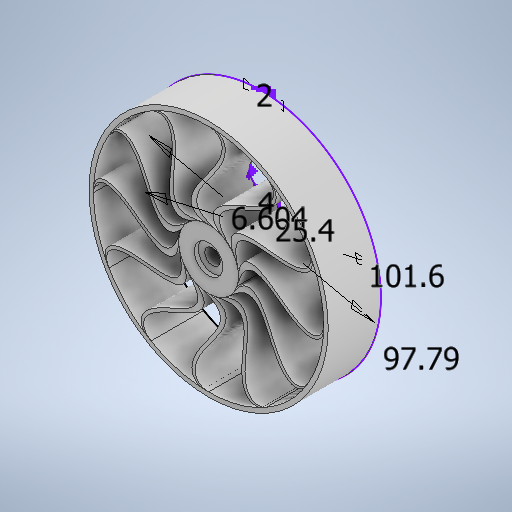
# Autodesk Inventor part: 12spoke_wheel
Saved by Autodesk Inventor 2025 (Build 290162000, 162)
## iProperties
Created: 2026-06-02
Part Number: 12spoke_wheel
Material: Generic
Document SubType Name: Modeling
Designer: localadmin
Density: 1 g/cm^3
Appearance: Default
Mass: 42.7852 g
Surface Area: 446.484 cm^2
Volume: 42.7852 cm^3
Author: localadmin
Autodesk Inventor part; units mm, degrees
ref_plane "YZ Plane" through (0, 0, 0) normal (1, 0, 0) x (0, 1, 0)
ref_plane "XZ Plane" through (0, 0, 0) normal (0, 1, 0) x (-1, 0, 0)
ref_plane "XY Plane" through (0, 0, 0) normal (0, 0, 1) x (1, 0, 0)
sketch "Sketch1" plane through (0, 0, 0) normal (0, 0, 1) x (1, 0, 0)
  circle A0 centre (0, 0) radius 48.895
  circle A1 centre (0, 0) radius 12.7
  circle A2 centre (0, 0) radius 3.302
  circle A3 centre (0, 0) radius 50.8
  spline S0 degree 4 poles (0.0017, 12.7) (-4.575, 12.7006) (-18.9819, 17.7432) (15.076, 40.8683) (4.6222, 48.8951) (-0.0006, 48.895) knots 0 0 0 0 0 0.502634 1 1 1 1 1
  spline S1 degree 4 poles (4.0017, 12.0531) (-0.7671, 13.6364) (-17.3734, 18.1808) (14.1216, 37.7355) (6.9874, 48.65) (1.9994, 48.8541) knots 0 0 0 0 0 0.509091 1 1 1 1 1
  point P0 (-8.0822, 8.0822)
  point P1 (-11.43, 0)
  point P2 (-8.0822, -8.0822)
  point P3 (0, -11.43)
  point P4 (8.0822, -8.0822)
  point P5 (11.43, 0)
  point P6 (8.0822, 8.0822)
  point P7 (0, 50.8)
  point P8 (-7.4232, 17.7252)
  point P9 (5.7258, 42.9245)
  point P10 (-5.0198, 19.0011)
  point P11 (6.8386, 41.5463)
  point P12 (4.0017, 12.0531)
  dimension "d19" = 101.6
  dimension "d0" = 97.79
  dimension "d2" = 25.4
  dimension "d14" = 6.604
  dimension "d61" = 2
  dimension "d62" = 4
  constraints: 4 point on circle, 3 centre point, 3 coincident, 1 vertical alignment, 14 other
  measures "d0" diameter of A0
  measures "d2" diameter of A1
  measures "d14" diameter of A2
  measures "d61" horizontal distance of A0.end A0.start
  measures "d62" horizontal distance of A1.end A1.start
extrude "Extrusion5" add sketch "Sketch1" along normal blind 22.4 contours S1 A1 S0 A0 picked at (-1.6908, 27.5381)
extrude "Extrusion1" add sketch "Sketch1" along normal blind 22.4 separate body contours A1 | A3
pattern_circular "Circular Pattern2" count 12 over 360 about axis through (0, 0, 0) along (0, 0, 1) bodies 2 1
sketch "Sketch5" plane through (0, 0, 0) normal (0, 0, -1) x (-1, 0, 0)
  circle A0 centre (0, 0) radius 6.1
  dimension "d52" = 12.2
  constraints: 1 centre point, 1 coincident
  measures "d52" diameter of A0
extrude "Extrusion3" cut sketch "Sketch5" against normal blind 1.7 bodies 2
sketch "Sketch6" plane through (0, 0, 22.4) normal (0, 0, 1) x (1, 0, 0)
  circle A0 centre (0, 0) radius 6.1
  constraints: 1 centre point, 1 coincident
extrude "Extrusion4" cut sketch "Sketch6" against normal blind 1.7018 bodies 2
body "Solid1"
body "Solid2"
